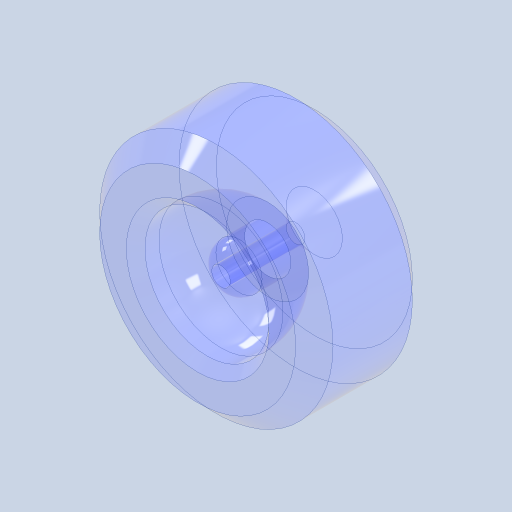
# Autodesk Inventor part: cpd_ultra-TLA100.3_0.7_stand_20230615
Saved by Autodesk Inventor 2024 (Build 280153000, 153)
## iProperties
Created: 2022-02-17
Part Number: cpd_ultra-TLA100.3_0.7_stand_20230615
Material: Generic
Document SubType Name: Modeling
Designer: to172
Density: 1 g/cm^3
Appearance: Clear - Blue
Author: to172
Autodesk Inventor part; units mm, degrees
ref_plane "YZ Plane" through (0, 0, 0) normal (1, 0, 0) x (0, 1, 0)
ref_plane "XZ Plane" through (0, 0, 0) normal (0, 1, 0) x (-1, 0, 0)
ref_plane "XY Plane" through (0, 0, 0) normal (0, 0, 1) x (1, 0, 0)
sketch "Sketch1" plane through (0, 0, 0) normal (0, 0, 1) x (1, 0, 0)
  line L0 (0, 0) -> (0, 18.187) construction
  line L1 (0, 0) -> (18.1544, 0) construction
  circle A0 centre (0, 0) radius 12.5
  circle A1 centre (0, 0) radius 2.475
  dimension "d0" = 25
  dimension "d24" = 4.95
  constraints: 4 end point, 2 centre point, 2 coincident, 1 horizontal, 1 vertical
  measures "d0" diameter of A0
  measures "d24" diameter of A1
extrude "Extrusion1" add sketch "Sketch1" along normal blind 5 contours A0 | A1
extrude "Extrusion2" add sketch "Sketch1" along normal blind 10 contours A1
sketch "Sketch2" plane through (0, 0, 0) normal (1, 0, 0) x (0, 1, 0)
  circle A0 centre (0, 10) radius 6.65
  line L0 (-6.65, 10) -> (-6.65, 12.5)
  line L1 (-6.65, 12.5) -> (-12.5, 12.5)
  line L2 (-12.5, 12.5) -> (-12.5, 5)
  line L3 (-12.5, 0) -> (-12.5, 5) projected
  line L4 (0, 10) -> (-27.2283, 10) construction
  line L5 (0, 3.35) -> (0, 5)
  line L6 (12.5, 5) -> (-12.5, 5) projected
  line L7 (0, 0) -> (0, 25) construction
  line L8 (0, 5) -> (-12.5, 5)
  line L9 (2.475, 10) -> (-2.475, 10) projected
  point P0 (-4.3843, 5)
  dimension "d8" = 13.3
  dimension "d9" = 2.5
  constraints: 14 end point, 3 perpendicular, 2 midpoint, 2 point on circle, 2 point on line, 2 vertical, 1 centre point, 1 collinear, 1 horizontal, 1 tangent
  measures "d8" diameter of A0
  measures "d9" distance between parallel lines of L1 L4
revolve "Revolution1" add sketch "Sketch2" angle 360 about axis through (0, 0, 0) along (0, 0, 1) contours A0 L6 L2 L1 L0
chamfer "Chamfer1" distance 2 angle 45 2 edges at (0, 12.5, 12.5) (-12.5, 0, 0)
chamfer "Chamfer2" distance 1 angle 45 1 edges at (0, 6.65, 12.5)
sketch "Sketch3" plane through (0, 0, 0) normal (0, 0, -1) x (-1, 0, 0)
  circle A0 centre (0, 0) radius 1
  dimension "d17" = 2
  constraints: 1 centre point, 1 coincident
  measures "d17" diameter of A0
extrude "Extrusion3" cut sketch "Sketch3" against normal through all
chamfer "Chamfer3" distance 2 angle 45 1 edges at (1, 0, 0)
fillet "Fillet1" radius 2 1 edges at (-2.475, 0, 10)
body "Solid1"
